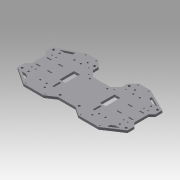
# Autodesk Inventor part: Support_Moteur
Saved by Autodesk Inventor 2016 (Build 200138000, 138)
## iProperties
Created: 2015-09-29
Part Number: Support_Moteur
Material: Générique
Document SubType Name: Modeling
Designer: Logan
Density: 1 g/cm^3
Appearance: Par défaut
Author: Logan
Autodesk Inventor part; units mm, degrees
ref_plane "YZ Plane" through (0, 0, 0) normal (1, 0, 0) x (0, 1, 0)
ref_plane "XZ Plane" through (0, 0, 0) normal (0, 1, 0) x (-1, 0, 0)
ref_plane "XY Plane" through (0, 0, 0) normal (0, 0, 1) x (1, 0, 0)
sketch "Esquisse1" plane through (0, 0, 0) normal (0, 0, 1) x (1, 0, 0)
  line L0 (-190, -60) -> (-190, 60)
  line L1 (190, 60) -> (190, -60)
  line L2 (-110, 100) -> (-190, 60)
  line L3 (110, 100) -> (190, 60)
  line L4 (-190, -60) -> (-130, -100)
  line L5 (130, -100) -> (190, -60)
  line L6 (70, 100) -> (110, 100)
  line L7 (130, -100) -> (60, -100)
  line L8 (-60, -100) -> (-130, -100)
  line L9 (30, 40) -> (-30, 40)
  line L10 (-110, 100) -> (-70, 100)
  line L11 (60, 100) -> (110, 100)
  line L12 (-60, -100) -> (-30, -80)
  line L13 (-30, -80) -> (30, -80)
  line L14 (30, -80) -> (60, -100)
  line L15 (-50, 60) -> (-50, 80)
  line L16 (50, 60) -> (50, 80)
  line L17 (-30, 40) -> (-50, 60)
  line L18 (30, 40) -> (50, 60)
  line L19 (-70, 100) -> (-50, 80)
  line L20 (70, 100) -> (50, 80)
  point P0 (0, 0)
  point P1 (-60, 100)
  point P2 (-50, 40)
  point P3 (50, 40)
  point P4 (-50, 100)
  point P5 (50, 100)
  dimension "d204" = 60
  dimension "d207" = 50
  dimension "d208" = 50
  dimension "d211" = 20
  dimension "d212" = 30
  dimension "d213" = 30
  dimension "d214" = 20
  dimension "d215" = 20
  dimension "d216" = 20
  dimension "d217" = 20
  dimension "d218" = 20
  dimension "d219" = 20
  dimension "d220" = 20
  dimension "d221" = 20
  dimension "d227" = 80
  dimension "d228" = 40
  dimension "d229" = 60
  dimension "d230" = 40
  dimension "d231" = 80
  dimension "d232" = 40
  dimension "d233" = 60
  dimension "d234" = 380
  dimension "d235" = 190
  dimension "d236" = 30
  dimension "d250" = 60
  dimension "d251" = 40
  constraints: 42 end point, 10 point on line, 7 parallel, 3 horizontal, 2 collinear, 2 perpendicular, 2 vertical
  measures "d204" distance between parallel lines of L9 L10
  measures "d207" horizontal distance of point (0, 0) point (50, 40)
  measures "d208" horizontal distance of point (0, 0) point (-50, 40)
  measures "d211" distance between parallel lines of L8 L13
  measures "d212" horizontal distance of L12.end L8.start
  measures "d213" horizontal distance of L7.end L13.end
  measures "d214" distance of L9.end point (-50, 40)
  measures "d215" distance of L15.start point (-50, 40)
  measures "d216" distance of L9.start point (50, 40)
  measures "d217" distance of L16.start point (50, 40)
  measures "d218" distance of L10.end point (-50, 100)
  measures "d219" distance of L15.end point (-50, 100)
  measures "d220" distance of L6.start point (50, 100)
  measures "d221" distance of L16.end point (50, 100)
  measures "d227" horizontal distance of L2.start L0.end
  measures "d228" vertical distance of L2.start L0.end
  measures "d229" horizontal distance of L0.start L4.end
  measures "d230" vertical distance of L0.start L4.end
  measures "d231" horizontal distance of L3.start L1.start
  measures "d232" vertical distance of L3.start L1.start
  measures "d233" distance of L12.end L13.end
  measures "d234" distance between parallel lines of L1 L0
  measures "d235" distance from line of point (0, 0) L0
  measures "d236" horizontal distance of point (0, 0) L13.end
  measures "d250" horizontal distance of L5.start L1.end
  measures "d251" vertical distance of L5.start L1.end
extrude "Plaque" add sketch "Esquisse1" along normal blind 8
sketch "Esquisse2" plane through (0, 0, 8) normal (0, 0, 1) x (1, 0, 0)
  circle A0 centre (-166, 35) radius 2
  circle A1 centre (-152, 35) radius 2
  circle A2 centre (-166, -35) radius 2
  circle A3 centre (-152, -35) radius 2
  line L0 (-190, 60) -> (-190, -60) projected
  line L1 (0, 25.5561) -> (0, -26.1527)
  circle A4 centre (166, 35) radius 2
  circle A5 centre (152, 35) radius 2
  circle A6 centre (166, -35) radius 2
  circle A7 centre (152, -35) radius 2
  point P0 (0, 0)
  dimension "d12" = 4
  dimension "d13" = 4
  dimension "d14" = 4
  dimension "d15" = 4
  dimension "d16" = 14
  dimension "d17" = 14
  dimension "d18" = 24
  dimension "d19" = 24
  dimension "d20" = 35
  dimension "d21" = 35
  dimension "d22" = 35
  dimension "d23" = 35
  constraints: 8 centre point, 4 symmetric about line, 2 end point, 1 vertical, 4 other
  measures "d12" diameter of A0
  measures "d13" diameter of A1
  measures "d14" diameter of A3
  measures "d15" diameter of A2
  measures "d16" distance of A1.centre A0.centre
  measures "d17" distance of A3.centre A2.centre
  measures "d18" distance from line of L0 A0.centre
  measures "d19" distance from line of L0 A2.centre
  measures "d20" vertical distance of point (0, 0) A2.centre
  measures "d21" vertical distance of point (0, 0) A3.centre
  measures "d22" vertical distance of point (0, 0) A1.centre
  measures "d23" vertical distance of point (0, 0) A0.centre
hole "Fixation_Encodeur" at (-152, 35, 8) at (-166, 35, 8) at (-166, -35, 8) at (-152, -35, 8) at (152, 35, 8) at (166, 35, 8) at (166, -35, 8) at (152, -35, 8) direction (0, 0, -1) diameter 4 end through all
sketch "Esquisse3" plane through (0, 0, 8) normal (0, 0, 1) x (1, 0, 0)
  line L0 (-120.5, -19) -> (-120.5, 19)
  line L1 (-160.5, 19) -> (-160.5, -19)
  line L2 (-160.5, -19) -> (-120.5, 19) construction
  line L3 (-120.5, -19) -> (-160.5, 19) construction
  line L4 (-110, 100) -> (-190, 60) projected
  line L5 (-190, 60) -> (-190, -60) projected
  line L6 (-190, -60) -> (-130, -100) projected
  line L7 (60, -100) -> (130, -100) projected
  line L8 (130, -100) -> (190, -60) projected
  line L9 (190, -60) -> (190, 60) projected
  line L10 (190, 60) -> (110, 100) projected
  line L11 (-70, 100) -> (-110, 100) projected
  line L12 (0, 102.1518) -> (0, -90)
  line L13 (-130, -100) -> (-60, -100) projected
  line L14 (30, 40) -> (-30, 40) projected
  line L15 (-60, -100) -> (-30, -80) projected
  line L16 (-30, -80) -> (30, -80) projected
  line L17 (30, -80) -> (60, -100) projected
  line L18 (70, 100) -> (50, 80) projected
  line L19 (50, 80) -> (50, 60) projected
  line L20 (50, 60) -> (30, 40) projected
  line L21 (-30, 40) -> (-50, 60) projected
  line L22 (-50, 60) -> (-50, 80) projected
  line L23 (-50, 80) -> (-70, 100) projected
  line L24 (110, 100) -> (70, 100) projected
  line L25 (-166.5, 19) -> (-154.5, 19)
  line L26 (-126.5, 19) -> (-114.5, 19)
  line L27 (-30, 0) -> (30, 0)
  line L28 (-166.5, 19) -> (-154.5, 19) construction
  line L29 (-166.5, 17) -> (-154.5, 17)
  line L30 (-154.5, 21) -> (-166.5, 21)
  arc A0 (-166.5, 21) -> (-166.5, 17) centre (-166.5, 19) ccw
  arc A1 (-154.5, 17) -> (-154.5, 21) centre (-154.5, 19) ccw
  line L31 (-126.5, 19) -> (-114.5, 19) construction
  line L32 (-126.5, 17) -> (-114.5, 17)
  line L33 (-114.5, 21) -> (-126.5, 21)
  arc A2 (-126.5, 21) -> (-126.5, 17) centre (-126.5, 19) ccw
  arc A3 (-114.5, 17) -> (-114.5, 21) centre (-114.5, 19) ccw
  line L34 (-166.5, -19) -> (-154.5, -19)
  line L35 (-126.5, -19) -> (-114.5, -19)
  line L36 (-166.5, -19) -> (-154.5, -19) construction
  line L37 (-166.5, -17) -> (-154.5, -17)
  line L38 (-154.5, -21) -> (-166.5, -21)
  arc A4 (-166.5, -17) -> (-166.5, -21) centre (-166.5, -19) ccw
  arc A5 (-154.5, -21) -> (-154.5, -17) centre (-154.5, -19) ccw
  line L39 (-126.5, -19) -> (-114.5, -19) construction
  line L40 (-126.5, -17) -> (-114.5, -17)
  line L41 (-114.5, -21) -> (-126.5, -21)
  arc A6 (-126.5, -17) -> (-126.5, -21) centre (-126.5, -19) ccw
  arc A7 (-114.5, -21) -> (-114.5, -17) centre (-114.5, -19) ccw
  line L42 (120.5, -19) -> (120.5, 19)
  line L43 (160.5, 19) -> (160.5, -19)
  line L44 (160.5, -19) -> (120.5, 19) construction
  line L45 (120.5, -19) -> (160.5, 19) construction
  line L46 (166.5, 19) -> (154.5, 19)
  line L47 (126.5, 19) -> (114.5, 19)
  line L48 (166.5, 19) -> (154.5, 19) construction
  line L49 (166.5, 17) -> (154.5, 17)
  line L50 (154.5, 21) -> (166.5, 21)
  arc A8 (166.5, 17) -> (166.5, 21) centre (166.5, 19) ccw
  arc A9 (154.5, 21) -> (154.5, 17) centre (154.5, 19) ccw
  line L51 (126.5, 19) -> (114.5, 19) construction
  line L52 (126.5, 17) -> (114.5, 17)
  line L53 (114.5, 21) -> (126.5, 21)
  arc A10 (126.5, 17) -> (126.5, 21) centre (126.5, 19) ccw
  arc A11 (114.5, 21) -> (114.5, 17) centre (114.5, 19) ccw
  arc A12 (154.5, -17) -> (154.5, -21) centre (154.5, -19) ccw
  line L54 (166.5, -19) -> (154.5, -19) construction
  line L55 (166.5, -19) -> (154.5, -19)
  line L56 (166.5, -17) -> (154.5, -17)
  arc A13 (166.5, -21) -> (166.5, -17) centre (166.5, -19) ccw
  line L57 (114.5, -21) -> (126.5, -21)
  line L58 (154.5, -21) -> (166.5, -21)
  line L59 (126.5, -17) -> (114.5, -17)
  line L60 (126.5, -19) -> (114.5, -19)
  line L61 (126.5, -19) -> (114.5, -19) construction
  arc A14 (114.5, -17) -> (114.5, -21) centre (114.5, -19) ccw
  arc A15 (126.5, -21) -> (126.5, -17) centre (126.5, -19) ccw
  point P0 (0, 0)
  point P1 (-140.5, 0)
  point P2 (-120.5, 19)
  point P3 (-160.5, -19)
  point P4 (-120.5, -19)
  point P5 (140.5, 0)
  point P6 (120.5, 19)
  point P7 (160.5, -19)
  point P8 (120.5, -19)
  dimension "d31" = 29.5
  dimension "d32" = 40
  dimension "d242" = 12
  dimension "d243" = 6
  dimension "d244" = 12
  dimension "d245" = 6
  dimension "d246" = 4
  dimension "d247" = 4
  constraints: 100 end point, 47 symmetric about line, 32 point on circle, 16 centre point, 14 midpoint, 8 tangent, 5 equal length, 2 horizontal, 1 vertical, 12 other
  measures "d31" distance between parallel lines of L5 L1
  measures "d32" distance between parallel lines of L1 L0
  measures "d242" distance of L25.start L25.end
  measures "d243" distance from line of L25.start L1
  measures "d244" distance of L26.start L26.end
  measures "d245" distance from line of L0 L26.end
  measures "d246" diameter of A1
  measures "d247" diameter of A3
extrude "Extrusion5" cut sketch "Esquisse3" against normal up to next contours L32 A2 L33 A3 | L40 A7 L41 A6 | L37 A5 L38 A4 | L29 A0 L30 A1 | L52 A11 L53 A10 | L59 A15 L57 A14 | L56 A13 L58 A12 | L49 A9 L50 A8
sketch "Esquisse4" plane through (0, 0, 8) normal (0, 0, 1) x (1, 0, 0)
  line L0 (-80, -25) -> (-60, -25)
  line L1 (-80, 25) -> (-80, -25)
  line L2 (-80, -25) -> (-59.915, 7.067) construction
  line L3 (-110, 100) -> (-190, 60) projected
  line L4 (-190, 60) -> (-190, -60) projected
  line L5 (-190, -60) -> (-130, -100) projected
  line L6 (60, -100) -> (130, -100) projected
  line L7 (130, -100) -> (190, -60) projected
  line L8 (190, -60) -> (190, 60) projected
  line L9 (190, 60) -> (110, 100) projected
  line L10 (-70, 100) -> (-110, 100) projected
  line L11 (60, 25) -> (80, 25)
  line L12 (80, 25) -> (80, -25)
  line L13 (80, -25) -> (60, -10.6364) construction
  line L14 (60, 25) -> (60, -25)
  line L15 (-60, -25) -> (-60, 25)
  line L16 (-60, 25) -> (-80, 25)
  line L17 (-59.915, 7.067) -> (-80, 25) construction
  line L18 (60, 10.0232) -> (80, 25) construction
  line L19 (80, -25) -> (60, -25)
  line L20 (-130, -100) -> (-60, -100) projected
  line L21 (30, 40) -> (-30, 40) projected
  line L22 (-60, -100) -> (-30, -80) projected
  line L23 (-30, -80) -> (30, -80) projected
  line L24 (30, -80) -> (60, -100) projected
  line L25 (70, 100) -> (50, 80) projected
  line L26 (50, 80) -> (50, 60) projected
  line L27 (50, 60) -> (30, 40) projected
  line L28 (-30, 40) -> (-50, 60) projected
  line L29 (-50, 60) -> (-50, 80) projected
  line L30 (-50, 80) -> (-70, 100) projected
  line L31 (110, 100) -> (70, 100) projected
  point P0 (-59.915, 7.067)
  dimension "d50" = 110
  dimension "d157" = 110
  dimension "d158" = 20
  dimension "d159" = 20
  constraints: 24 end point, 3 point on line, 2 collinear, 2 parallel, 1 horizontal
  measures "d50" distance between parallel lines of L4 L1
  measures "d157" distance between parallel lines of L8 L12
  measures "d158" distance between parallel lines of L1 L15
  measures "d159" distance between parallel lines of L12 L14
extrude "Passage_Courroie" cut sketch "Esquisse4" against normal up to surface (8 mm away) contours L1 L16 L15 L0 | L11 L12 L19 L14
sketch "Esquisse5" plane through (0, 0, 8) normal (0, 0, 1) x (1, 0, 0)
  line L0 (0, 30.4597) -> (0, -30.4597)
  line L1 (-17.5456, 0) -> (17.5456, 0)
  line L2 (-158, 53.1115) -> (-116.2229, 74)
  line L3 (-116.2229, 74) -> (-82, 74)
  line L4 (-82, 74) -> (-82, -74)
  line L5 (-82, -74) -> (-129.1054, -74)
  line L6 (-129.1054, -74) -> (-158, -54.4961)
  line L7 (116.2229, 74) -> (82, 74)
  line L8 (158, 53.1115) -> (116.2229, 74)
  line L9 (82, -74) -> (129.1054, -74)
  line L10 (129.1054, -74) -> (158, -54.4961)
  line L11 (-190, 60) -> (-190, -60) projected
  point P0 (0, 0)
  point P1 (0, 0)
  dimension "d175" = 47.1054
  dimension "d176" = 34.2229
  dimension "d177" = 41.7771
  dimension "d178" = 28.8946
  dimension "d179" = 32
  dimension "d180" = 32
  dimension "d240" = 148
  constraints: 22 end point, 6 symmetric about line, 2 midpoint, 2 vertical, 1 coincident, 1 horizontal
  measures "d175" distance of L4.end L5.end
  measures "d176" distance of L3.start L3.end
  measures "d177" horizontal distance of L2.start L3.start
  measures "d178" horizontal distance of L5.end L6.end
  measures "d179" distance from line of L11 L6.end
  measures "d180" distance from line of L11 L2.start
  measures "d240" distance of L3.end L4.end
hole "Fixation_Base" at (158, 53.1115, 8) at (82, 74, 8) at (158, -54.4961, 8) at (82, -74, 8) at (-82, -74, 8) at (-158, -54.4961, 8) at (-158, 53.1115, 8) at (-82, 74, 8) direction (0, 0, -1) diameter 6 end through all
sketch "Esquisse8" plane through (0, 0, 8) normal (0, 0, 1) x (1, 0, 0)
  line L0 (-178, -30) -> (-190, -30)
  line L1 (-190, -30) -> (-190, 30)
  line L2 (-190, 30) -> (-178, 30)
  line L3 (-178, 30) -> (-178, -30)
  line L4 (-178, -30) -> (-190, 30) construction
  line L5 (-190, -30) -> (-178, 30) construction
  line L6 (0, 43.7993) -> (0, -83.0015)
  line L7 (178, -30) -> (190, -30)
  line L8 (190, -30) -> (190, 30)
  line L9 (190, 30) -> (178, 30)
  line L10 (178, 30) -> (178, -30)
  line L11 (178, -30) -> (190, 30) construction
  line L12 (190, -30) -> (178, 30) construction
  point P0 (0, 0)
  point P1 (-184, 0)
  point P2 (184, 0)
  dimension "d106" = 60
  dimension "d107" = 12
  dimension "d108" = 178
  dimension "d191" = 30
  constraints: 26 end point, 5 symmetric about line, 4 midpoint, 2 parallel, 1 horizontal, 1 perpendicular, 1 vertical
  measures "d106" distance of L2.end L0.start
  measures "d107" distance of L1.end L2.end
  measures "d108" distance from line of point (0, 0) L3
  measures "d191" distance from line of point (0, 0) L2
extrude "Passage_Encodeur" cut sketch "Esquisse8" against normal up to surface (8 mm away)
chamfer "Passage_cable" distance 6 angle 45 8 edges at (-178, 30, 4) (-178, -30, 4) (178, 30, 4) (178, -30, 4) (190, 30, 4) (-190, 30, 4) (-190, -30, 4) (190, -30, 4)
sketch "Esquisse10" plane through (0, 0, 8) normal (0, 0, 1) x (1, 0, 0)
  line L0 (-70, -35) -> (-70, -55) construction
  line L1 (-73, -35) -> (-73, -55)
  line L2 (-67, -55) -> (-67, -35)
  arc A0 (-67, -35) -> (-73, -35) centre (-70, -35) ccw
  arc A1 (-73, -55) -> (-67, -55) centre (-70, -55) ccw
  line L3 (-60, -25) -> (-80, -25) projected
  line L4 (0, 0) -> (0, -51.7085)
  line L5 (70, -35) -> (70, -55) construction
  line L6 (73, -35) -> (73, -55)
  line L7 (67, -55) -> (67, -35)
  arc A2 (73, -35) -> (67, -35) centre (70, -35) ccw
  arc A3 (67, -55) -> (73, -55) centre (70, -55) ccw
  point P0 (-70, -45)
  point P1 (70, -45)
  dimension "d192" = 10
  dimension "d193" = 20
  dimension "d194" = 3
  dimension "d195" = 10
  constraints: 18 end point, 8 point on circle, 7 symmetric about line, 4 centre point, 4 tangent, 2 vertical, 1 midpoint, 1 parallel, 2 other
  measures "d192" distance from line of L3 L0.start
  measures "d193" distance of L0.start L0.end
  measures "d194" distance from line of point (-70, -45) L2
  measures "d195" horizontal distance of L3.end point (-70, -45)
extrude "Fixation_Galet" cut sketch "Esquisse10" against normal blind 10
sketch "Esquisse11" plane through (0, 0, 8) normal (0, 0, 1) x (1, 0, 0)
  line L0 (0, 0) -> (0, -70.3583)
  line L1 (-113, 59) -> (-91, 59)
  line L2 (-91, 59) -> (-91, -59)
  line L3 (-91, -59) -> (-113, -59)
  line L4 (-113, -59) -> (-113, 59)
  line L5 (-80, -25) -> (-80, 25) projected
  line L6 (113, 59) -> (91, 59)
  line L7 (91, 59) -> (91, -59)
  line L8 (91, -59) -> (113, -59)
  line L9 (113, -59) -> (113, 59)
  dimension "d252" = 118
  dimension "d253" = 59
  dimension "d254" = 22
  dimension "d255" = 11
  constraints: 18 end point, 4 symmetric about line, 2 parallel, 1 horizontal, 1 perpendicular, 1 vertical
  measures "d252" distance between parallel lines of L3 L1
  measures "d253" distance from line of L0.start L3
  measures "d254" distance between parallel lines of L2 L4
  measures "d255" distance between parallel lines of L5 L2
hole "Suport_Wheel" at (-113, 59, 8) at (-91, 59, 8) at (-113, -59, 8) at (-91, -59, 8) at (91, -59, 8) at (113, -59, 8) at (113, 59, 8) at (91, 59, 8) direction (0, 0, -1) diameter 6 end through all
sketch "Esquisse12" plane through (0, 0, 8) normal (0, 0, 1) x (1, 0, 0)
  circle A0 centre (113, 59) radius 3 projected
  circle A1 centre (91, -59) radius 3 projected
  circle A2 centre (-113, -59) radius 3 projected
  circle A3 centre (-113, 59) radius 3 projected
  circle A4 centre (-91, 59) radius 3 projected
  circle A5 centre (-91, -59) radius 3 projected
  circle A6 centre (113, -59) radius 3 projected
  circle A7 centre (91, 59) radius 3 projected
  arc A8 (-73, -55) -> (-67, -55) centre (-70, -55) ccw projected
  line L0 (-73, -55) -> (-73, -35) projected
  arc A9 (-67, -35) -> (-73, -35) centre (-70, -35) ccw projected
  line L1 (-67, -35) -> (-67, -55) projected
  arc A10 (73, -35) -> (67, -35) centre (70, -35) ccw projected
  line L2 (73, -35) -> (73, -55) projected
  arc A11 (67, -55) -> (73, -55) centre (70, -55) ccw projected
  line L3 (67, -55) -> (67, -35) projected
  line L4 (178, -24) -> (190, -36) projected
  line L5 (178, -24) -> (178, 24) projected
  line L6 (190, 36) -> (178, 24) projected
  line L7 (190, 36) -> (190, 60) projected
  line L8 (190, 60) -> (110, 100) projected
  line L9 (110, 100) -> (70, 100) projected
  line L10 (70, 100) -> (50, 80) projected
  line L11 (50, 80) -> (50, 60) projected
  line L12 (50, 60) -> (30, 40) projected
  line L13 (30, 40) -> (-30, 40) projected
  line L14 (-30, 40) -> (-50, 60) projected
  line L15 (-50, 60) -> (-50, 80) projected
  line L16 (-50, 80) -> (-70, 100) projected
  line L17 (-70, 100) -> (-110, 100) projected
  line L18 (-110, 100) -> (-190, 60) projected
  line L19 (-190, 60) -> (-190, 36) projected
  line L20 (-178, 24) -> (-190, 36) projected
  line L21 (-178, 24) -> (-178, -24) projected
  line L22 (-190, -36) -> (-178, -24) projected
  line L23 (-190, -36) -> (-190, -60) projected
  line L24 (-190, -60) -> (-130, -100) projected
  line L25 (-130, -100) -> (-60, -100) projected
  line L26 (-60, -100) -> (-30, -80) projected
  line L27 (-30, -80) -> (30, -80) projected
  line L28 (30, -80) -> (60, -100) projected
  line L29 (60, -100) -> (130, -100) projected
  line L30 (130, -100) -> (190, -60) projected
  line L31 (190, -60) -> (190, -36) projected
  circle A12 centre (-158, 53.1115) radius 3 projected
  circle A13 centre (-82, -74) radius 3 projected
  circle A14 centre (158, -54.4961) radius 3 projected
  circle A15 centre (158, 53.1115) radius 3 projected
  circle A16 centre (82, 74) radius 3 projected
  circle A17 centre (82, -74) radius 3 projected
  circle A18 centre (-158, -54.4961) radius 3 projected
  circle A19 centre (-82, 74) radius 3 projected
  line L32 (80, 25) -> (80, -25) projected
  line L33 (80, -25) -> (60, -25) projected
  line L34 (60, -25) -> (60, 25) projected
  line L35 (60, 25) -> (80, 25) projected
  line L36 (-80, -25) -> (-80, 25) projected
  line L37 (-80, 25) -> (-60, 25) projected
  line L38 (-60, 25) -> (-60, -25) projected
  line L39 (-60, -25) -> (-80, -25) projected
  arc A20 (166.5, 17) -> (166.5, 21) centre (166.5, 19) ccw projected
  line L40 (166.5, 17) -> (154.5, 17) projected
  arc A21 (154.5, 21) -> (154.5, 17) centre (154.5, 19) ccw projected
  line L41 (154.5, 21) -> (166.5, 21) projected
  arc A22 (114.5, 21) -> (114.5, 17) centre (114.5, 19) ccw projected
  line L42 (114.5, 21) -> (126.5, 21) projected
  arc A23 (126.5, 17) -> (126.5, 21) centre (126.5, 19) ccw projected
  line L43 (126.5, 17) -> (114.5, 17) projected
  arc A24 (-166.5, -17) -> (-166.5, -21) centre (-166.5, -19) ccw projected
  line L44 (-166.5, -17) -> (-154.5, -17) projected
  arc A25 (-154.5, -21) -> (-154.5, -17) centre (-154.5, -19) ccw projected
  line L45 (-154.5, -21) -> (-166.5, -21) projected
  arc A26 (-154.5, 17) -> (-154.5, 21) centre (-154.5, 19) ccw projected
  line L46 (-154.5, 17) -> (-166.5, 17) projected
  arc A27 (-166.5, 21) -> (-166.5, 17) centre (-166.5, 19) ccw projected
  line L47 (-166.5, 21) -> (-154.5, 21) projected
  arc A28 (-114.5, 17) -> (-114.5, 21) centre (-114.5, 19) ccw projected
  line L48 (-114.5, 17) -> (-126.5, 17) projected
  arc A29 (-126.5, 21) -> (-126.5, 17) centre (-126.5, 19) ccw projected
  line L49 (-126.5, 21) -> (-114.5, 21) projected
  arc A30 (-114.5, -21) -> (-114.5, -17) centre (-114.5, -19) ccw projected
  line L50 (-114.5, -21) -> (-126.5, -21) projected
  arc A31 (-126.5, -17) -> (-126.5, -21) centre (-126.5, -19) ccw projected
  line L51 (-126.5, -17) -> (-114.5, -17) projected
  arc A32 (126.5, -21) -> (126.5, -17) centre (126.5, -19) ccw projected
  line L52 (126.5, -21) -> (114.5, -21) projected
  arc A33 (114.5, -17) -> (114.5, -21) centre (114.5, -19) ccw projected
  line L53 (114.5, -17) -> (126.5, -17) projected
  arc A34 (154.5, -17) -> (154.5, -21) centre (154.5, -19) ccw projected
  line L54 (154.5, -17) -> (166.5, -17) projected
  arc A35 (166.5, -21) -> (166.5, -17) centre (166.5, -19) ccw projected
  line L55 (166.5, -21) -> (154.5, -21) projected
  circle A36 centre (166, -35) radius 2 projected
  circle A37 centre (152, 35) radius 2 projected
  circle A38 centre (-166, -35) radius 2 projected
  circle A39 centre (-152, 35) radius 2 projected
  circle A40 centre (-166, 35) radius 2 projected
  circle A41 centre (-152, -35) radius 2 projected
  circle A42 centre (166, 35) radius 2 projected
  circle A43 centre (152, -35) radius 2 projected
  line L56 (-180, 53.8197) -> (-107.6393, 90)
  line L57 (-107.6393, 90) -> (-74.1421, 90)
  line L58 (-74.1421, 90) -> (-60, 75.8579)
  line L59 (-60, 75.8579) -> (-60, 55.8579)
  line L60 (-60, 55.8579) -> (-34.1421, 30)
  line L61 (-34.1421, 30) -> (34.1421, 30)
  line L62 (34.1421, 30) -> (60, 55.8579)
  line L63 (60, 55.8579) -> (60, 75.8579)
  line L64 (60, 75.8579) -> (74.1421, 90)
  line L65 (74.1421, 90) -> (107.6393, 90)
  line L66 (107.6393, 90) -> (180, 53.8197)
  line L67 (180, 53.8197) -> (180, 40.1421)
  line L68 (180, 40.1421) -> (168, 28.1421)
  line L69 (168, 28.1421) -> (168, -28.1421)
  line L70 (168, -28.1421) -> (180, -40.1421)
  line L71 (180, -40.1421) -> (180, -54.6482)
  line L72 (180, -54.6482) -> (126.9722, -90)
  line L73 (126.9722, -90) -> (63.0278, -90)
  line L74 (63.0278, -90) -> (33.0278, -70)
  line L75 (33.0278, -70) -> (-33.0278, -70)
  line L76 (-33.0278, -70) -> (-63.0278, -90)
  line L77 (-63.0278, -90) -> (-126.9722, -90)
  line L78 (-126.9722, -90) -> (-180, -54.6482)
  line L79 (-180, -54.6482) -> (-180, -40.1421)
  line L80 (-180, -40.1421) -> (-168, -28.1421)
  line L81 (-168, -28.1421) -> (-168, 28.1421)
  line L82 (-168, 28.1421) -> (-180, 40.1421)
  line L83 (-180, 40.1421) -> (-180, 53.8197)
  point P0 (0, 0)
  dimension "d263" = 10
  constraints: 56 end point, 27 other
  measures "d263" distance between parallel lines of L18 L56
hole "Support_Etage" at (-180, 53.8197, 8) at (180, 53.8197, 8) at (180, -54.6482, 8) at (-180, -54.6482, 8) at (-60, 75.8579, 8) at (60, 75.8579, 8) at (33.0278, -70, 8) at (-33.0278, -70, 8) direction (0, 0, -1) diameter 8 end through all
sketch "Esquisse13" plane through (0, 0, 8) normal (0, 0, 1) x (1, 0, 0)
  line L0 (64.1421, 60) -> (44.1421, 40)
  line L1 (-44.1421, 40) -> (-64.1421, 60)
  line L2 (-30, 40) -> (-50, 60) projected
  line L3 (-30, 40) -> (-50, 60) projected
  line L4 (50, 60) -> (30, 40) projected
  point P0 (0, 0)
  dimension "d281" = 10
  dimension "d282" = 0
  dimension "d283" = 0
  dimension "d284" = 10
  dimension "d285" = 0
  dimension "d286" = 0
  constraints: 4 end point, 2 parallel
  measures "d281" distance between parallel lines of L2 L1
  measures "d282" vertical distance of L2.end L1.end
  measures "d283" vertical distance of L2.start L1.start
  measures "d284" distance between parallel lines of L4 L0
  measures "d285" vertical distance of L0.start L4.start
  measures "d286" vertical distance of L4.end L0.end
hole "Support_Guide" at (-64.1421, 60, 8) at (-44.1421, 40, 8) at (44.1421, 40, 8) at (64.1421, 60, 8) direction (0, 0, -1) diameter 4 end through all
sketch "Esquisse14" plane through (0, 0, 8) normal (0, 0, 1) x (1, 0, 0)
  line L0 (30, 40) -> (-30, 40) projected
  line L1 (30, 30) -> (-30, 30)
  point P0 (0, 0)
  dimension "d294" = 10
  constraints: 2 end point, 1 parallel
  measures "d294" distance between parallel lines of L0 L1
hole "Support_Elevateur" at (-30, 30, 8) at (30, 30, 8) direction (0, 0, -1) diameter 6 end through all
sketch "Esquisse15" plane through (0, 0, 8) normal (0, 0, 1) x (1, 0, 0)
  circle A0 centre (-30, 30) radius 3 projected
  circle A1 centre (30, 30) radius 3 projected
  circle A2 centre (44.1421, 40) radius 2 projected
  circle A3 centre (-64.1421, 60) radius 2 projected
  circle A4 centre (-44.1421, 40) radius 2 projected
  circle A5 centre (64.1421, 60) radius 2 projected
  circle A6 centre (33.0278, -70) radius 4 projected
  circle A7 centre (-60, 75.8579) radius 4 projected
  circle A8 centre (180, -54.6482) radius 4 projected
  circle A9 centre (-180, 53.8197) radius 4 projected
  circle A10 centre (180, 53.8197) radius 4 projected
  circle A11 centre (-180, -54.6482) radius 4 projected
  circle A12 centre (60, 75.8579) radius 4 projected
  circle A13 centre (-33.0278, -70) radius 4 projected
  circle A14 centre (113, 59) radius 3 projected
  circle A15 centre (91, -59) radius 3 projected
  circle A16 centre (-113, -59) radius 3 projected
  circle A17 centre (-113, 59) radius 3 projected
  circle A18 centre (-91, 59) radius 3 projected
  circle A19 centre (-91, -59) radius 3 projected
  circle A20 centre (113, -59) radius 3 projected
  circle A21 centre (91, 59) radius 3 projected
  arc A22 (-73, -55) -> (-67, -55) centre (-70, -55) ccw projected
  line L0 (-73, -55) -> (-73, -35) projected
  arc A23 (-67, -35) -> (-73, -35) centre (-70, -35) ccw projected
  line L1 (-67, -35) -> (-67, -55) projected
  arc A24 (73, -35) -> (67, -35) centre (70, -35) ccw projected
  line L2 (73, -35) -> (73, -55) projected
  arc A25 (67, -55) -> (73, -55) centre (70, -55) ccw projected
  line L3 (67, -55) -> (67, -35) projected
  line L4 (178, -24) -> (190, -36) projected
  line L5 (178, -24) -> (178, 24) projected
  line L6 (190, 36) -> (178, 24) projected
  line L7 (190, 36) -> (190, 60) projected
  line L8 (190, 60) -> (110, 100) projected
  line L9 (110, 100) -> (70, 100) projected
  line L10 (70, 100) -> (50, 80) projected
  line L11 (50, 80) -> (50, 60) projected
  line L12 (50, 60) -> (30, 40) projected
  line L13 (30, 40) -> (-30, 40) projected
  line L14 (-30, 40) -> (-50, 60) projected
  line L15 (-50, 60) -> (-50, 80) projected
  line L16 (-50, 80) -> (-70, 100) projected
  line L17 (-70, 100) -> (-110, 100) projected
  line L18 (-110, 100) -> (-190, 60) projected
  line L19 (-190, 60) -> (-190, 36) projected
  line L20 (-178, 24) -> (-190, 36) projected
  line L21 (-178, 24) -> (-178, -24) projected
  line L22 (-190, -36) -> (-178, -24) projected
  line L23 (-190, -36) -> (-190, -60) projected
  line L24 (-190, -60) -> (-130, -100) projected
  line L25 (-130, -100) -> (-60, -100) projected
  line L26 (-60, -100) -> (-30, -80) projected
  line L27 (-30, -80) -> (30, -80) projected
  line L28 (30, -80) -> (60, -100) projected
  line L29 (60, -100) -> (130, -100) projected
  line L30 (130, -100) -> (190, -60) projected
  line L31 (190, -60) -> (190, -36) projected
  circle A26 centre (-158, 53.1115) radius 3 projected
  circle A27 centre (-82, -74) radius 3 projected
  circle A28 centre (158, -54.4961) radius 3 projected
  circle A29 centre (158, 53.1115) radius 3 projected
  circle A30 centre (82, 74) radius 3 projected
  circle A31 centre (82, -74) radius 3 projected
  circle A32 centre (-158, -54.4961) radius 3 projected
  circle A33 centre (-82, 74) radius 3 projected
  line L32 (80, 25) -> (80, -25) projected
  line L33 (80, -25) -> (60, -25) projected
  line L34 (60, -25) -> (60, 25) projected
  line L35 (60, 25) -> (80, 25) projected
  line L36 (-80, -25) -> (-80, 25) projected
  line L37 (-80, 25) -> (-60, 25) projected
  line L38 (-60, 25) -> (-60, -25) projected
  line L39 (-60, -25) -> (-80, -25) projected
  arc A34 (166.5, 17) -> (166.5, 21) centre (166.5, 19) ccw projected
  line L40 (166.5, 17) -> (154.5, 17) projected
  arc A35 (154.5, 21) -> (154.5, 17) centre (154.5, 19) ccw projected
  line L41 (154.5, 21) -> (166.5, 21) projected
  arc A36 (114.5, 21) -> (114.5, 17) centre (114.5, 19) ccw projected
  line L42 (114.5, 21) -> (126.5, 21) projected
  arc A37 (126.5, 17) -> (126.5, 21) centre (126.5, 19) ccw projected
  line L43 (126.5, 17) -> (114.5, 17) projected
  arc A38 (-166.5, -17) -> (-166.5, -21) centre (-166.5, -19) ccw projected
  line L44 (-166.5, -17) -> (-154.5, -17) projected
  arc A39 (-154.5, -21) -> (-154.5, -17) centre (-154.5, -19) ccw projected
  line L45 (-154.5, -21) -> (-166.5, -21) projected
  arc A40 (-154.5, 17) -> (-154.5, 21) centre (-154.5, 19) ccw projected
  line L46 (-154.5, 17) -> (-166.5, 17) projected
  arc A41 (-166.5, 21) -> (-166.5, 17) centre (-166.5, 19) ccw projected
  line L47 (-166.5, 21) -> (-154.5, 21) projected
  arc A42 (-114.5, 17) -> (-114.5, 21) centre (-114.5, 19) ccw projected
  line L48 (-114.5, 17) -> (-126.5, 17) projected
  arc A43 (-126.5, 21) -> (-126.5, 17) centre (-126.5, 19) ccw projected
  line L49 (-126.5, 21) -> (-114.5, 21) projected
  arc A44 (-114.5, -21) -> (-114.5, -17) centre (-114.5, -19) ccw projected
  line L50 (-114.5, -21) -> (-126.5, -21) projected
  arc A45 (-126.5, -17) -> (-126.5, -21) centre (-126.5, -19) ccw projected
  line L51 (-126.5, -17) -> (-114.5, -17) projected
  arc A46 (126.5, -21) -> (126.5, -17) centre (126.5, -19) ccw projected
  line L52 (126.5, -21) -> (114.5, -21) projected
  arc A47 (114.5, -17) -> (114.5, -21) centre (114.5, -19) ccw projected
  line L53 (114.5, -17) -> (126.5, -17) projected
  arc A48 (154.5, -17) -> (154.5, -21) centre (154.5, -19) ccw projected
  line L54 (154.5, -17) -> (166.5, -17) projected
  arc A49 (166.5, -21) -> (166.5, -17) centre (166.5, -19) ccw projected
  line L55 (166.5, -21) -> (154.5, -21) projected
  circle A50 centre (166, -35) radius 2 projected
  circle A51 centre (152, 35) radius 2 projected
  circle A52 centre (-166, -35) radius 2 projected
  circle A53 centre (-152, 35) radius 2 projected
  circle A54 centre (-166, 35) radius 2 projected
  circle A55 centre (-152, -35) radius 2 projected
  circle A56 centre (166, 35) radius 2 projected
  circle A57 centre (152, -35) radius 2 projected
  line L56 (-108.5836, 94) -> (-72.4853, 94)
  line L57 (-72.4853, 94) -> (-56, 77.5147)
  line L58 (-56, 77.5147) -> (-56, 57.5147)
  line L59 (-56, 57.5147) -> (-32.4853, 34)
  line L60 (-32.4853, 34) -> (32.4853, 34)
  line L61 (32.4853, 34) -> (56, 57.5147)
  line L62 (56, 57.5147) -> (56, 77.5147)
  line L63 (56, 77.5147) -> (72.4853, 94)
  line L64 (72.4853, 94) -> (108.5836, 94)
  line L65 (108.5836, 94) -> (184, 56.2918)
  line L66 (184, 56.2918) -> (184, 38.4853)
  line L67 (184, 38.4853) -> (172, 26.4853)
  line L68 (172, 26.4853) -> (172, -26.4853)
  line L69 (172, -26.4853) -> (184, -38.4853)
  line L70 (184, -38.4853) -> (184, -56.7889)
  line L71 (184, -56.7889) -> (128.1833, -94)
  line L72 (128.1833, -94) -> (61.8167, -94)
  line L73 (61.8167, -94) -> (31.8167, -74)
  line L74 (31.8167, -74) -> (-31.8167, -74)
  line L75 (-31.8167, -74) -> (-61.8167, -94)
  line L76 (-61.8167, -94) -> (-128.1833, -94)
  line L77 (-128.1833, -94) -> (-184, -56.7889)
  line L78 (-184, -56.7889) -> (-184, -38.4853)
  line L79 (-184, -38.4853) -> (-172, -26.4853)
  line L80 (-172, -26.4853) -> (-172, 26.4853)
  line L81 (-172, 26.4853) -> (-184, 38.4853)
  line L82 (-184, 38.4853) -> (-184, 56.2918)
  line L83 (-184, 56.2918) -> (-108.5836, 94)
  point P0 (0, 0)
  dimension "d302" = 6
  constraints: 56 end point, 27 other
  measures "d302" distance between parallel lines of L17 L56
hole "Support_GP2" at (-108.5836, 94, 8) at (-72.4853, 94, 8) at (72.4853, 94, 8) at (108.5836, 94, 8) at (61.8167, -94, 8) at (128.1833, -94, 8) at (-61.8167, -94, 8) at (-128.1833, -94, 8) direction (0, 0, -1) diameter 4 end through all
sketch "Esquisse16" plane through (0, 0, 8) normal (0, 0, 1) x (1, 0, 0)
  line L0 (-110, 100) -> (-190, 60) projected
  line L1 (-169.9266, 63.3285) -> (-132.3607, 82.1115)
  line L2 (-132.3607, 82.1115) -> (-132.3607, 82.1115)
  line L3 (-132.3607, 73.1672) -> (-152.0381, 63.3285)
  line L4 (-169.9266, 63.3285) -> (-169.9266, 63.3285)
  line L5 (-132.3607, 82.1115) -> (-132.3607, 73.1672)
  line L6 (-152.0381, 63.3285) -> (-169.9266, 63.3285)
  line L7 (-50, 60) -> (-50, 80) projected
  line L8 (-70, 100) -> (-110, 100) projected
  line L9 (-190, -60) -> (-130, -100) projected
  line L10 (-169.9266, -66.1711) -> (-143.301, -83.9216)
  line L11 (-143.301, -83.9216) -> (-143.301, -83.9216)
  line L12 (-143.301, -74.3068) -> (-155.5044, -66.1711)
  line L13 (-169.9266, -66.1711) -> (-169.9266, -66.1711)
  line L14 (-155.5044, -66.1711) -> (-169.9266, -66.1711)
  line L15 (-143.301, -83.9216) -> (-143.301, -74.3068)
  line L16 (-190, -36) -> (-190, -60) projected
  line L17 (-130, -100) -> (-60, -100) projected
  line L18 (0, 0) -> (0, -41.1993)
  line L19 (110, 100) -> (190, 60)
  line L20 (169.9266, 63.3285) -> (132.3607, 82.1115)
  line L21 (132.3607, 82.1115) -> (132.3607, 82.1115)
  line L22 (132.3607, 73.1672) -> (152.0381, 63.3285)
  line L23 (169.9266, 63.3285) -> (169.9266, 63.3285)
  line L24 (132.3607, 82.1115) -> (132.3607, 73.1672)
  line L25 (152.0381, 63.3285) -> (169.9266, 63.3285)
  line L26 (50, 60) -> (50, 80)
  line L27 (70, 100) -> (110, 100)
  line L28 (190, -60) -> (130, -100)
  line L29 (169.9266, -66.1711) -> (143.301, -83.9216)
  line L30 (143.301, -83.9216) -> (143.301, -83.9216)
  line L31 (143.301, -74.3068) -> (155.5044, -66.1711)
  line L32 (169.9266, -66.1711) -> (169.9266, -66.1711)
  line L33 (155.5044, -66.1711) -> (169.9266, -66.1711)
  line L34 (143.301, -83.9216) -> (143.301, -74.3068)
  line L35 (190, -36) -> (190, -60)
  line L36 (130, -100) -> (60, -100)
  point P0 (-128.783, 74.956)
  point P1 (-166.3489, 56.1731)
  point P2 (-138.8634, -77.2652)
  point P3 (-165.489, -59.5147)
  point P4 (128.783, 74.956)
  point P5 (166.3489, 56.1731)
  point P6 (138.8634, -77.2652)
  point P7 (165.489, -59.5147)
  dimension "d310" = 8
  dimension "d311" = 6
  dimension "d312" = 42
  dimension "d313" = 28
  dimension "d316" = 8
  dimension "d319" = 8
  dimension "d320" = 8
  dimension "d323" = 32
  dimension "d324" = 6
  dimension "d326" = 8
  dimension "d327" = 8
  dimension "d329" = 0
  constraints: 62 end point, 25 symmetric about line, 16 point on line, 10 parallel, 2 perpendicular, 1 vertical
  measures "d310" distance between parallel lines of L1 L3
  measures "d311" distance between parallel lines of L0 L1
  measures "d312" distance between parallel lines of L2 L4
  measures "d313" distance from line of L0.start L2
  measures "d316" distance of L2.end point (-128.783, 74.956)
  measures "d319" distance of L4.start point (-166.349, 56.173)
  measures "d320" distance between parallel lines of L12 L10
  measures "d323" distance between parallel lines of L11 L13
  measures "d324" distance between parallel lines of L9 L10
  measures "d326" distance of L13.start point (-165.489, -59.515)
  measures "d327" distance of L11.end point (-138.863, -77.265)
  measures "d329" horizontal distance of L1.start L10.start
extrude "Extrusion6" cut sketch "Esquisse16" against normal up to next
